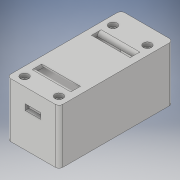
# Autodesk Inventor part: bottom
Saved by Autodesk Inventor 2017.3 (Build 213257000, 257)
## iProperties
Part Number: bottom
Material: Generisch
Document SubType Name: Modeling
Designer: Enno
Density: 1 g/cm^3
Appearance: Vorgabe
Author: Enno
Autodesk Inventor part; units mm, degrees
ref_plane "YZ Plane" through (0, 0, 0) normal (1, 0, 0) x (0, 1, 0)
ref_plane "XZ Plane" through (0, 0, 0) normal (0, 1, 0) x (-1, 0, 0)
ref_plane "XY Plane" through (0, 0, 0) normal (0, 0, 1) x (1, 0, 0)
sketch "Skizze1" plane through (0, 0, 0) normal (0, 0, 1) x (1, 0, 0)
  line L0 (0, 0) -> (27, 0)
  line L1 (27, 0) -> (27, 59)
  line L2 (27, 59) -> (0, 59)
  line L3 (0, 59) -> (0, 0)
  dimension "d0" = 27
  dimension "d1" = 59
  constraints: 8 end point, 2 parallel, 1 horizontal, 1 perpendicular
  measures "d0" distance of L1.end L2.end
  measures "d1" distance of L0.end L1.end
extrude "Extrusion1" add sketch "Skizze1" against normal blind 28.2
sketch "Skizze2" plane through (0, 0, -28.2) normal (0, 0, -1) x (-1, 0, 0)
  line L0 (-2, 57) -> (-25, 57)
  line L1 (-25, 57) -> (-25, 2)
  line L2 (-25, 2) -> (-2, 2)
  line L3 (-2, 2) -> (-2, 57)
  line L4 (0, 59) -> (-27, 59) construction
  line L5 (-27, 59) -> (-27, 0) construction
  point P0 (0, 0)
  dimension "d4" = 2
  dimension "d5" = 2
  dimension "d6" = 2
  dimension "d7" = 2
  constraints: 8 end point, 2 parallel, 1 horizontal, 1 perpendicular
  measures "d4" distance from line of point (0, 0) L2
  measures "d5" distance from line of point (0, 0) L3
  measures "d6" distance from line of L4 L0.start
  measures "d7" distance from line of L5 L0.end
extrude "Extrusion2" cut sketch "Skizze2" against normal blind 26.2
sketch "Skizze3" plane through (0, 0, -2) normal (0, 0, -1) x (-1, 0, 0)
  circle A0 centre (-4.61, 4.57) radius 3
  line L0 (-2, 2) -> (-25, 2) construction
  line L1 (-2, 57) -> (-2, 2) construction
  circle A1 centre (-22.39, 4.57) radius 3
  circle A2 centre (-4.61, 50.29) radius 3
  circle A3 centre (-22.39, 50.29) radius 3
  line L2 (-4.61, 4.57) -> (-22.39, 4.57) construction
  point P0 (0, 0)
  point P1 (-13.5, 4.57)
  point P2 (-13.5, 2)
  dimension "d13" = 6
  dimension "d18" = 17.78
  dimension "d21" = 45.72
  dimension "d66" = 2.57
  constraints: 4 centre point, 2 end point, 2 horizontal, 2 midpoint, 1 vertical, 1 vertical alignment, 6 other
  measures "d13" diameter of A0
  measures "d18" distance of L2.start L2.end
  measures "d21" distance of L2.start A2.centre
  measures "d66" distance from line of L0 L2.start
extrude "Extrusion4" add sketch "Skizze3" along normal blind 3.5
sketch "Skizze7" plane through (4.61, 50.29, -5.5) normal (0, 0, -1) x (0, -1, 0)
  circle A0 centre (0, 0) radius 3 construction
  circle A1 centre (0, -17.78) radius 3 construction
  circle A2 centre (45.72, -17.78) radius 3 construction
  circle A3 centre (45.72, 0) radius 3 construction
  point P0 (50.29, 4.61)
  point P1 (0, -17.78)
  point P2 (45.72, 0)
  constraints: 4 coincident
hole "Bohrung2" at (4.61, 50.29, -5.5) at (22.39, 50.29, -5.5) at (22.39, 4.57, -5.5) at (4.61, 4.57, -5.5) direction (0, 0, 1) diameter 2.5 end through all
sketch "Skizze8" plane through (0, 0, -2) normal (0, 0, -1) x (-1, 0, 0)
  line L0 (-3.5, 11.57) -> (-23.5, 11.57)
  line L1 (-23.5, 11.57) -> (-23.5, 14.57)
  line L2 (-23.5, 14.57) -> (-3.5, 14.57)
  line L3 (-3.5, 14.57) -> (-3.5, 11.57)
  line L4 (-2, 2) -> (-25, 2) construction
  circle A0 centre (-4.61, 4.57) radius 3 construction
  line L5 (-3.5, 43.29) -> (-23.5, 43.29)
  line L6 (-23.5, 43.29) -> (-23.5, 40.29)
  line L7 (-23.5, 40.29) -> (-3.5, 40.29)
  line L8 (-3.5, 40.29) -> (-3.5, 43.29)
  circle A1 centre (-4.61, 50.29) radius 3 construction
  point P0 (0, 0)
  point P1 (-13.5, 11.57)
  point P2 (-13.5, 2)
  point P3 (-13.5, 2)
  point P4 (-13.5, 40.29)
  dimension "d43" = 3
  dimension "d44" = 20
  dimension "d45" = 4
  dimension "d46" = 3
  dimension "d47" = 20
  dimension "d48" = 4
  constraints: 16 end point, 4 midpoint, 4 parallel, 2 horizontal, 2 perpendicular, 2 vertical alignment
  measures "d43" distance of L2.end L0.start
  measures "d44" distance of L0.start L0.end
  measures "d45" distance edge to line of A0 L0
  measures "d46" distance of L7.end L5.start
  measures "d47" distance of L6.end L7.end
  measures "d48" distance edge to line of A1 L5
extrude "Extrusion5" cut sketch "Skizze8" against normal through all
sketch "Skizze9" plane through (0, 0, 0) normal (0, -1, 0) x (1, 0, 0)
  line L0 (2, -5.5) -> (3.0624, -5.5) construction
  line L1 (17.5, -10.5) -> (9.5, -10.5)
  line L2 (9.5, -10.5) -> (9.5, -7.5)
  line L3 (9.5, -7.5) -> (17.5, -7.5)
  line L4 (17.5, -7.5) -> (17.5, -10.5)
  line L5 (0, 0) -> (27, 0) construction
  point P0 (13.5, -7.5)
  point P1 (13.5, 0)
  dimension "d54" = 8
  dimension "d55" = 3
  dimension "d56" = 2
  constraints: 8 end point, 2 midpoint, 2 parallel, 1 horizontal, 1 perpendicular, 1 vertical alignment
  measures "d54" distance of L2.end L3.end
  measures "d55" distance of L1.end L2.end
  measures "d56" distance between parallel lines of L3 L0
extrude "Extrusion6" cut sketch "Skizze9" against normal up to surface (2 mm away)
sketch "Skizze10" plane through (0, 0, 0) normal (0, 0, 1) x (1, 0, 0)
  circle A0 centre (4.61, 4.57) radius 1.25 construction
  circle A1 centre (22.39, 4.57) radius 1.25 construction
  circle A2 centre (22.39, 50.29) radius 1.25 construction
  circle A3 centre (4.61, 50.29) radius 1.25 construction
  point P0 (0, 0)
  constraints: 4 coincident
hole "Bohrung3" at (4.61, 4.57, 0) at (22.39, 4.57, 0) at (22.39, 50.29, 0) at (4.61, 50.29, 0) direction (0, 0, -1) diameter 2.5 end through all counterbore diameter 4.2 counterbore depth 2
fillet "Rundung1" radius 2 4 edges at (27, 0, -14.1) (0, 0, -14.1) (0, 59, -14.1) (27, 59, -14.1)
fillet "Rundung2" radius 2 2 edges at (13.5, 14.57, -2) (13.5, 40.29, -2)
fillet "Rundung3" radius 2 2 edges at (13.5, 11.57, 0) (13.5, 43.29, 0)
